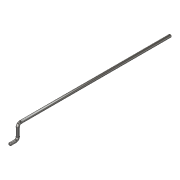
# Autodesk Inventor part: AILERON
Saved by Autodesk Inventor 2019 (Build 230136000, 136)
## iProperties
Created: 2022-04-05
Part Number: AILERON
Material: Steel, High Strength, Low Alloy
Document SubType Name: Modeling
Designer: solyo
Density: 7.85 g/cm^3
Appearance: Steel - Polished
Mass: 0.383126 g
Surface Area: 1.96794 cm^2
Volume: 0.0488059 cm^3
Author: solyo
Autodesk Inventor part; units mm, degrees
ref_plane "YZ Plane" through (0, 0, 0) normal (1, 0, 0) x (0, 1, 0)
ref_plane "XZ Plane" through (0, 0, 0) normal (0, 1, 0) x (-1, 0, 0)
ref_plane "XY Plane" through (0, 0, 0) normal (0, 0, 1) x (1, 0, 0)
sketch "Sketch1" plane through (0, 0, 0) normal (0, 0, 1) x (1, 0, 0)
  circle A0 centre (0, 0) radius 0.5
  dimension "d0" = 1
  constraints: 1 centre point, 1 coincident
  measures "d0" diameter of A0
sketch "Sketch2" plane through (0, 0, 0) normal (1, 0, 0) x (0, 1, 0)
  line L0 (0, 0) -> (0, -2)
  line L1 (1, -3) -> (4, -3)
  line L2 (5, -4) -> (5, -58)
  arc A0 (5, -4) -> (4, -3) centre (4, -4) ccw
  arc A1 (0, -2) -> (1, -3) centre (1, -2) ccw
  point P0 (0, -3)
  point P1 (5, -3)
  dimension "d1" = 3
  dimension "d2" = 5
  dimension "d3" = 55
  dimension "d4" = 1
  constraints: 6 end point, 4 point on circle, 4 point on line, 4 tangent, 2 centre point, 2 perpendicular, 1 equal radius, 1 vertical
  measures "d1" distance of L0.start point (0, -3)
  measures "d2" distance of point (0, -3) point (5, -3)
  measures "d3" distance of point (5, -3) L2.end
  measures "d4" radius of A0
sweep "Sweep1" add profiles "Sketch1" path "Sketch2" path curves L0 A1 L1 A0 L2
chamfer "Chamfer1" distance 0.2 angle 45 2 edges at (-0.5, 0, 0) (-0.5, 5, -58)
equation "\"d3\" = Length"
equation "\"Length\" = 55"
body "Solid1"
